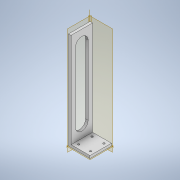
# Autodesk Inventor part: IDOM_infrared_fixture2
Saved by Autodesk Inventor 2022 (Build 260153000, 153)
## iProperties
Created: 2022-07-06
Part Number: IDOM_infrared_fixture2
Material: Generic
Document SubType Name: Modeling
Designer: dovalle
Density: 1 g/cm^3
Appearance: Default
Author: dovalle
Autodesk Inventor part; units mm, degrees
sketch "Sketch1" plane through (0, 0, 0) normal (0, 0, 1) x (1, 0, 0)
  line L0 (0, 0) -> (34, 0)
  line L1 (34, 0) -> (34, 4)
  line L2 (34, 4) -> (4, 4)
  line L3 (4, 4) -> (4, 154)
  line L4 (4, 154) -> (0, 154)
  line L5 (0, 154) -> (0, 0)
  dimension "d2" = 34
  dimension "d3" = 4
  dimension "d4" = 30
  dimension "d5" = 150
  dimension "d6" = 4
  constraints: 12 end point, 3 perpendicular, 1 horizontal, 1 vertical
  measures "d2" distance of L0.start L0.end
  measures "d3" distance of L0.end L1.end
  measures "d4" distance of L1.end L2.end
  measures "d5" distance of L2.end L3.end
  measures "d6" distance of L3.end L4.end
extrude "Extrusion1" add sketch "Sketch1" along normal blind 34
sketch "Sketch2" plane through (0, 0, 0) normal (0, -1, 0) x (1, 0, 0)
  line L0 (0, 0) -> (34, 0) projected
  line L1 (34, 0) -> (34, 34) projected
  line L2 (0, 34) -> (34, 34) projected
  line L3 (0, 0) -> (0, 34) projected
  line L4 (34, 0) -> (4, 0) projected
  line L5 (4, 0) -> (4, 34) projected
  line L6 (34, 34) -> (4, 34) projected
  line L7 (34, 0) -> (34, 34) projected
  line L8 (34, 0) -> (34, 34) projected
  line L9 (34, 34) -> (4, 34) projected
  circle A0 centre (9.6433, 27.6042) radius 1.5
  circle A1 centre (28.3567, 27.6042) radius 1.5
  circle A2 centre (28.3567, 6.3958) radius 1.5
  circle A3 centre (9.6433, 6.3958) radius 1.5
  dimension "d10" = 3
  dimension "d11" = 3
  dimension "d12" = 3
  dimension "d13" = 3
  constraints: 4 centre point
  measures "d10" diameter of A0
  measures "d11" diameter of A1
  measures "d12" diameter of A2
  measures "d13" diameter of A3
extrude "Extrusion2" cut sketch "Sketch2" against normal blind 20 contours A0 | A1 | A2 | A3
sketch "Sketch3" plane through (4, 4, 0) normal (1, 0, 0) x (0, 0, -1)
  line L0 (0, 0) -> (-34, 0) projected
  line L1 (0, 150) -> (-34, 150) projected
  arc A0 (-27, 20) -> (-7, 20) centre (-17, 20) ccw
  arc A1 (-7, 130) -> (-27, 130) centre (-17, 130) ccw
  line L2 (-27, 20) -> (-27, 130)
  line L3 (-7, 130) -> (-7, 20)
  point P0 (0, -4)
  constraints: 4 end point, 4 point on circle, 2 centre point, 2 vertical
extrude "Extrusion3" cut sketch "Sketch3" against normal blind 20
body "Solid1"
